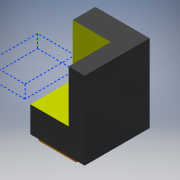
# Autodesk Inventor part: part_a
Saved by Autodesk Inventor 2019 (Build 230136000, 136)
## iProperties
Created: 2019-01-14
Part Number: part_a
Material: Generic
Document SubType Name: Modeling
Designer: jmc
Density: 1 g/cm^3
Appearance: Dark Gray
Author: jmc
Autodesk Inventor part; units mm, degrees
ref_plane "YZ Plane" through (0, 0, 0) normal (1, 0, 0) x (0, 1, 0)
ref_plane "XZ Plane" through (0, 0, 0) normal (0, 1, 0) x (-1, 0, 0)
ref_plane "XY Plane" through (0, 0, 0) normal (0, 0, 1) x (1, 0, 0)
sketch "Sketch1" plane through (0, 0, 0) normal (0, 1, 0) x (-1, 0, 0)
  line L0 (9.597, 9.7392) -> (-11.3031, 9.7392)
  line L1 (-11.3031, 9.7392) -> (-11.3031, -15.2841)
  line L2 (-11.3031, -15.2841) -> (9.597, -15.2841)
  line L3 (9.597, -15.2841) -> (9.597, 9.7392)
  point P0 (0, 0)
  constraints: 8 end point, 2 parallel, 1 horizontal, 1 perpendicular
extrude "Extrusion1" add sketch "Sketch1" along normal blind 30
sketch "Sketch2" plane through (0, 30, 0) normal (0, 1, 0) x (1, 0, 0)
  line L0 (-9.597, -9.7392) -> (11.3031, -9.7392) projected
  line L1 (-9.597, -9.7392) -> (5.1013, -9.7392)
  line L2 (5.1013, -9.7392) -> (5.1013, 6.5588)
  line L3 (5.1013, 6.5588) -> (-9.597, 6.5588)
  line L4 (-9.597, 6.5588) -> (-9.597, -9.7392)
  point P0 (0, 0)
  constraints: 8 end point, 2 parallel, 1 horizontal, 1 perpendicular
extrude "Extrusion2" cut sketch "Sketch2" against normal blind 20
sketch "Sketch4" plane through (0, 0, 0) normal (0, -1, 0) x (1, 0, 0)
  line L0 (6.1052, -11.4334) -> (-8.3253, -11.4334)
  line L1 (-8.3253, -11.4334) -> (-8.3253, 7.8258)
  line L2 (-8.3253, 7.8258) -> (6.1052, 7.8258)
  line L3 (6.1052, 7.8258) -> (6.1052, -11.4334)
  point P0 (0, 0)
  constraints: 8 end point, 2 parallel, 1 horizontal, 1 perpendicular
extrude "Extrusion4" add sketch "Sketch4" along normal mid plane 5 separate body
body "Solid1"
body "Solid3"
